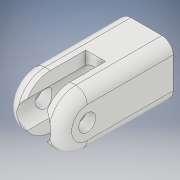
# Autodesk Inventor part: Arm6
Saved by Autodesk Inventor 2017 SP1 (Build 210196100, 196)
## iProperties
Created: 2018-02-11
Part Number: Arm6
Material: ABS Plastic
Document SubType Name: Modeling
Designer: Zach
Density: 1.06 g/cm^3
Appearance: CR White
Author: Zach
Autodesk Inventor part; units mm, degrees
ref_plane "YZ Plane" through (0, 0, 0) normal (1, 0, 0) x (0, 1, 0)
ref_plane "XZ Plane" through (0, 0, 0) normal (0, 1, 0) x (-1, 0, 0)
ref_plane "XY Plane" through (0, 0, 0) normal (0, 0, 1) x (1, 0, 0)
sketch "Sketch1" plane through (0, 0, 0) normal (0, 0, 1) x (1, 0, 0)
  line L0 (0, 0) -> (9.5, 0)
  line L1 (9.5, 0) -> (9.5, 9.5)
  line L2 (9.5, 9.5) -> (0, 9.5)
  line L3 (0, 9.5) -> (0, 0)
  dimension "d0" = 9.5
  dimension "d1" = 9.5
  constraints: 8 end point, 2 parallel, 1 horizontal, 1 perpendicular
  measures "d0" distance of L2.end L1.end
  measures "d1" distance of L1.end L0.end
extrude "Extrusion1" add sketch "Sketch1" along normal blind 9
sketch "Sketch2" plane through (9.5, 0, 0) normal (1, 0, 0) x (0, 0, -1)
  circle A0 centre (-15.25, 4.75) radius 4.75 construction
  line L0 (0, 0) -> (0, 9.5) projected
  line L1 (-9, 0) -> (-9, 9.5) projected
  line L2 (-9, 9.5) -> (-15.25, 9.5)
  line L3 (-9, 0) -> (-15.25, 0)
  arc A1 (-15.25, 9.5) -> (-15.25, 0) centre (-15.25, 4.75) ccw
  circle A2 centre (-15.25, 4.75) radius 1.5
  point P0 (0, 4.75)
  point P1 (0, 4.75)
  dimension "d4" = 9.5
  dimension "d5" = 15.25
  dimension "d6" = 3
  constraints: 4 end point, 4 point on circle, 3 centre point, 2 midpoint, 2 tangent, 1 coincident, 1 horizontal alignment, 1 parallel
  measures "d4" diameter of A0
  measures "d5" distance from line of L0 A0.centre
  measures "d6" diameter of A2
extrude "Extrusion2" add sketch "Sketch2" against normal blind 3
sketch "Sketch3" plane through (0, 0, 0) normal (-1, 0, 0) x (0, 0, 1)
  circle A0 centre (15.25, 4.75) radius 1.5 projected
  line L0 (9, 0) -> (9, 9.5) projected
  line L1 (9, 0) -> (15.25, 0) projected
  arc A1 (15.25, 0) -> (15.25, 9.5) centre (15.25, 4.75) ccw projected
  line L2 (15.25, 9.5) -> (9, 9.5) projected
  point P0 (0, 0)
extrude "Extrusion3" add sketch "Sketch3" against normal blind 3
fillet "Fillet1" radius 2 6 edges at (0, 4.75, 20) (0, 0, 7.625) (0, 9.5, 7.625) (9.5, 4.75, 20) (9.5, 0, 7.625) (9.5, 9.5, 7.625)
sketch "Sketch4" plane through (0, 0, 0) normal (0, 0, -1) x (-1, 0, 0)
  circle A0 centre (-4.75, 4.75) radius 2
  line L0 (-7.5, 9.5) -> (-2, 9.5) projected
  line L1 (0, 7.5) -> (0, 2) projected
  point P0 (0, 0)
  point P1 (0, 4.75)
  point P2 (-4.75, 9.5)
  dimension "d12" = 4
  constraints: 2 midpoint, 1 centre point, 1 horizontal alignment, 1 vertical alignment
  measures "d12" diameter of A0
extrude "Extrusion4" cut sketch "Sketch4" against normal through all
sketch "Sketch5" plane through (0, 0, 9) normal (0, 0, 1) x (1, 0, 0)
  circle A0 centre (4.75, 4.75) radius 2 projected
  circle A1 centre (4.75, 4.75) radius 3
  point P0 (0, 0)
  dimension "d15" = 6
  constraints: 1 centre point, 1 coincident
  measures "d15" diameter of A1
extrude "Extrusion5" cut sketch "Sketch5" along normal blind 15 and the other way blind 6
body "Solid1"
